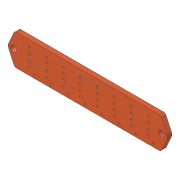
# Autodesk Inventor part: IMUTrackerBase_8port_hub_pcb
Saved by Autodesk Inventor 2019.4 (Build 234330000, 330)
## iProperties
Created: 2019-11-19
Part Number: IMUTrackerBase_8port_hub_pcb
Material: 一般
Document SubType Name: Modeling
Designer: y6tada
Density: 1 g/cm^3
Appearance: 滑らか - 淡いオレンジ
Author: y6tada
Autodesk Inventor part; units mm, degrees
ref_plane "YZ Plane" through (0, 0, 0) normal (1, 0, 0) x (0, 1, 0)
ref_plane "XZ Plane" through (0, 0, 0) normal (0, 1, 0) x (-1, 0, 0)
ref_plane "XY Plane" through (0, 0, 0) normal (0, 0, 1) x (1, 0, 0)
sketch "スケッチ1" plane through (0, 0, 0) normal (0, 0, 1) x (1, 0, 0)
  circle A0 centre (-26.15, 0) radius 1.1
  circle A1 centre (-20.55, 3) radius 0.4
  circle A2 centre (-18.85, 4.5) radius 0.4 construction
  circle A3 centre (-20.55, 1) radius 0.4
  circle A4 centre (-20.55, -1) radius 0.4
  circle A5 centre (-20.55, -3) radius 0.4
  circle A6 centre (-14.55, 3) radius 0.4
  circle A7 centre (-12.85, 4.5) radius 0.4 construction
  circle A8 centre (-14.55, 1) radius 0.4
  circle A9 centre (-14.55, -1) radius 0.4
  circle A10 centre (-14.55, -3) radius 0.4
  circle A11 centre (-8.55, 3) radius 0.4
  circle A12 centre (-6.85, 4.5) radius 0.4 construction
  circle A13 centre (-8.55, 1) radius 0.4
  circle A14 centre (-8.55, -1) radius 0.4
  circle A15 centre (-8.55, -3) radius 0.4
  circle A16 centre (-2.55, 3) radius 0.4
  circle A17 centre (-0.85, 4.5) radius 0.4 construction
  circle A18 centre (-2.55, 1) radius 0.4
  circle A19 centre (-2.55, -1) radius 0.4
  circle A20 centre (-2.55, -3) radius 0.4
  circle A21 centre (3.45, 3) radius 0.4
  circle A22 centre (5.15, 4.5) radius 0.4 construction
  circle A23 centre (3.45, 1) radius 0.4
  circle A24 centre (3.45, -1) radius 0.4
  circle A25 centre (3.45, -3) radius 0.4
  circle A26 centre (9.45, 3) radius 0.4
  circle A27 centre (11.15, 4.5) radius 0.4 construction
  circle A28 centre (9.45, 1) radius 0.4
  circle A29 centre (9.45, -1) radius 0.4
  circle A30 centre (9.45, -3) radius 0.4
  circle A31 centre (15.45, 3) radius 0.4
  circle A32 centre (17.15, 4.5) radius 0.4 construction
  circle A33 centre (15.45, 1) radius 0.4
  circle A34 centre (15.45, -1) radius 0.4
  circle A35 centre (15.45, -3) radius 0.4
  circle A36 centre (21.45, 3) radius 0.4
  circle A37 centre (23.15, 4.5) radius 0.4 construction
  circle A38 centre (21.45, 1) radius 0.4
  circle A39 centre (21.45, -1) radius 0.4
  circle A40 centre (21.45, -3) radius 0.4
  line L0 (-26.1134, -4.9138) -> (-27.9707, -0.8276)
  arc A41 (-27.9707, 0.8276) -> (-27.9707, -0.8276) centre (-26.15, 0) ccw
  line L1 (-27.9707, 0.8276) -> (-26.1134, 4.9138)
  arc A42 (-25.203, 5.5) -> (-26.1134, 4.9138) centre (-25.203, 4.5) ccw
  line L2 (-25.203, 5.5) -> (25.203, 5.5)
  arc A43 (26.1134, 4.9138) -> (25.203, 5.5) centre (25.203, 4.5) ccw
  line L3 (26.1134, 4.9138) -> (27.9707, 0.8276)
  arc A44 (27.9707, -0.8276) -> (27.9707, 0.8276) centre (26.15, 0) ccw
  line L4 (27.9707, -0.8276) -> (26.1134, -4.9138)
  arc A45 (25.203, -5.5) -> (26.1134, -4.9138) centre (25.203, -4.5) ccw
  line L5 (25.203, -5.5) -> (-25.203, -5.5)
  arc A46 (-26.1134, -4.9138) -> (-25.203, -5.5) centre (-25.203, -4.5) ccw
  circle A47 centre (26.15, 0) radius 1.1
  line L6 (-26.15, 0) -> (26.15, 0) construction
  line L7 (0, 0) -> (0, 14.1732) construction
  circle A48 centre (-18.85, -4.5) radius 0.4
  circle A49 centre (-12.85, -4.5) radius 0.4
  circle A50 centre (-6.85, -4.5) radius 0.4
  circle A51 centre (-0.85, -4.5) radius 0.4
  circle A52 centre (5.15, -4.5) radius 0.4
  circle A53 centre (11.15, -4.5) radius 0.4
  circle A54 centre (17.15, -4.5) radius 0.4
  circle A55 centre (23.15, -4.5) radius 0.4
  constraints: 56 centre point, 43 equal radius, 16 end point, 12 point on circle, 12 symmetric about line, 12 tangent, 4 horizontal, 2 vertical, 1 midpoint, 122 other
extrude "押し出し1" add sketch "スケッチ1" along normal blind 1.6
